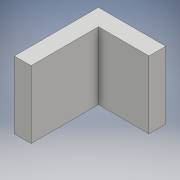
# Autodesk Inventor part: Esteira - Carro
Saved by Autodesk Inventor 2017 (Build 210142000, 142)
## iProperties
Created: 2020-09-19
Part Number: Esteira - Carro
Material: Generic
Document SubType Name: Modeling
Designer: ale
Density: 1 g/cm^3
Appearance: Default
Author: ale
Autodesk Inventor part; units mm, degrees
ref_plane "YZ Plane" through (0, 0, 0) normal (1, 0, 0) x (0, 1, 0)
ref_plane "XZ Plane" through (0, 0, 0) normal (0, 1, 0) x (-1, 0, 0)
ref_plane "XY Plane" through (0, 0, 0) normal (0, 0, 1) x (1, 0, 0)
sketch "Sketch1" plane through (0, 0, 0) normal (0, 0, 1) x (1, 0, 0)
  line L0 (0, -20) -> (0, 0)
  line L1 (0, 0) -> (15, 0)
  line L2 (-5, -20) -> (-5, 5)
  line L3 (-5, 5) -> (15, 5)
  line L4 (0, -20) -> (-5, -20)
  line L5 (15, 5) -> (15, 0)
  dimension "d0" = 15
  dimension "d1" = 20
  dimension "d2" = 5
  constraints: 12 end point, 3 perpendicular, 1 horizontal, 1 vertical, 1 other
  measures "d0" distance of L0.end L1.end
  measures "d1" distance of L0.start L0.end
  measures "d2" distance between parallel lines of L0 L2
extrude "Extrusion1" add sketch "Sketch1" along normal blind 20
body "Solid1"
